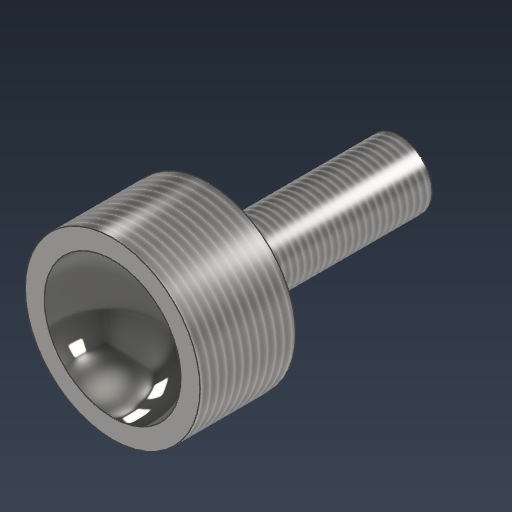
# Autodesk Inventor part: MCEN4000:T1
Saved by Autodesk Inventor 2021 (Build 250183000, 183)
## iProperties
Created: 2020-10-15
Part Number: MCEN4000:T1
Material: STEEL, AISI 1040
Document SubType Name: Modeling
Designer: Eugene Tang
Mass: 109.446 g
Surface Area: 51.7813 cm^2
Volume: 13.9421 cm^3
Density: 7.85 g/cm^3
Appearance: Semi-Polished(1)
Description: TIE ROD INNER CUP
dv: 1.083 mm
dvBigDIA: 0.135 mm
dt: 0.768 mm
dvSmallDIA: 0.128 mm
MinorDIA: 12.000 mm
Pitch: 1.250 mm
a: 0.052 mm
BallJointBall_Dia: 25.000 mm
BallJointBody_THICKNESS: 3.500 mm
BodyDepth: 5.000 mm
q: 40.000 mm
d84: 32.000 mm
Author: Eugene Tang
Autodesk Inventor part; units mm, degrees
ref_plane "YZ Plane" through (0, 0, 0) normal (1, 0, 0) x (0, 1, 0)
ref_plane "XZ Plane" through (0, 0, 0) normal (0, 1, 0) x (-1, 0, 0)
ref_plane "XY Plane" through (0, 0, 0) normal (0, 0, 1) x (1, 0, 0)
sketch "Sketch1" plane through (0, 0, 0) normal (0, 0, 1) x (1, 0, 0)
  circle A0 centre (0, 0) radius 13
  dimension "d0" = 26
  constraints: 1 centre point, 1 coincident
  measures "d0" diameter of A0
sketch "Sketch2" plane through (0, 0, 0) normal (0, 0, 1) x (1, 0, 0)
  circle A0 centre (0, 0) radius 6
  dimension "MinorDIA" = 12
  constraints: 1 centre point, 1 coincident
  measures "MinorDIA" diameter of A0
extrude "Extrusion1" add sketch "Sketch2" against normal blind 40
sketch "Sketch4" plane through (0, 0, 0) normal (1, 0, 0) x (0, 1, 0)
  line L0 (0, 0) -> (0, 25) construction
  circle A0 centre (0, 12.5) radius 12.5 construction
  line L1 (6, 0) -> (-6, 0) projected
  line L2 (6, 0) -> (-6, 0) projected
  line L3 (-16, 12.5) -> (-12.5, 12.5)
  line L4 (-16, 12.5) -> (-16, -5)
  line L5 (-16, -5) -> (0, -5)
  line L6 (0, -5) -> (0, 0)
  line L7 (-12.5, 27.5) -> (-12.5, -3.4028) construction
  arc A1 (-12.5, 12.5) -> (0, 0) centre (0, 12.5) ccw
  dimension "BallJointBall_Dia" = 25
  dimension "BodyDepth" = 5
  dimension "BallJointBody_THICKNESS" = 3.5
  dimension "d52" = 17.5
  constraints: 12 end point, 4 point on circle, 3 tangent, 3 vertical, 2 centre point, 2 perpendicular, 1 horizontal, 1 midpoint, 1 point on line
  measures "BallJointBall_Dia" diameter of A0
  measures "BodyDepth" distance between parallel lines of L5 L1
  measures "BallJointBody_THICKNESS" distance between parallel lines of L4 L7
  measures "d52" distance between parallel lines of L5 L3
revolve "Revolution1" add sketch "Sketch4" angle 360 about axis through (0, 0, 0) along (0, 0, 1)
sketch "Sketch5" plane through (0, 0, 0) normal (1, 0, 0) x (0, 1, 0)
  line L0 (-6, -40) -> (6, -40) construction
  line L1 (6, -40) -> (6, -47.8199) construction
  line L2 (7.0825, -39.5608) -> (7.0825, -47.5953) construction
  line L3 (6.9472, -42.5792) -> (6.9472, -40) construction
  line L4 (6.1797, -43.2466) -> (6.1797, -39.9527) construction
  line L5 (7.0825, -40.625) -> (6, -40.625) construction
  line L6 (6.1279, -41.25) -> (6.1279, -40) construction
  line L7 (6, -40) -> (7.0825, -40) construction
  line L8 (6, -41.25) -> (7.0825, -41.25) construction
  line L9 (7.0825, -40) -> (6, -40.625) construction
  line L10 (6, -40.625) -> (7.0825, -41.25) construction
  arc A0 (6.1797, -40.5213) -> (6.1797, -40.7287) centre (6.2578, -40.625) ccw
  line L11 (6.9472, -40) -> (6.9472, -40.0781)
  line L12 (6.9472, -40.0781) -> (6.1797, -40.5213)
  line L13 (6.9472, -41.1719) -> (6.9472, -41.25)
  line L14 (6.9472, -41.1719) -> (6.1797, -40.7287)
  line L15 (6.9472, -40.0781) -> (6.9472, -41.1719)
  point P0 (0, 0)
  dimension "dv" = 1.0825
  dimension "dvBigDIA" = 0.1353
  dimension "dt" = 0.7675
  dimension "d12" = 1.25
  dimension "d13" = 0.625
  dimension "dvSmallDIA" = 0.1279
  dimension "d16" = 0.9472
  dimension "d19" = 59.999
  dimension "d22" = 0.5469
  dimension "a" = 0.0518
  constraints: 30 end point, 18 point on line, 3 perpendicular, 3 vertical, 2 collinear, 2 parallel, 2 point on circle, 1 centre point, 1 tangent
  measures "dv" distance between parallel lines of L1 L2
  measures "dvBigDIA" distance between parallel lines of L2 L3
  measures "dt" distance between parallel lines of L3 L4
  measures "d12" distance of L0.end L8.start
  measures "d13" distance from line of L8.start L5
  measures "dvSmallDIA" distance between parallel lines of L6 L1
  measures "d16" distance between parallel lines of L3 L1
  measures "d19" angle of L1 L9
  measures "d22" distance from line of L11.end L5
  measures "a" distance between parallel lines of L6 L4
thread "Thread5" size "M12x1.25" class "6g" standard "ISO Metric profile" full length
thread "Thread6" size "M32x1.5" class "6g" standard "ISO Metric profile" full length
sketch "Sketch13" plane through (0, 0, 12.5) normal (0, 0, 1) x (1, 0, 0)
  circle A0 centre (0, 0) radius 16 projected
  dimension "d84" = 32
  measures "d84" diameter of A0
equation "\"d0\" = SteeringColumn_DIA"
equation "\"dv\" = 0.866 * Pitch"
equation "\"dvBigDIA\" = 0.125 * dv"
equation "\"dt\" = 0.614 * Pitch"
equation "\"d12\" = Pitch"
equation "\"d13\" = 0.5 * d12"
equation "\"dvSmallDIA\" = 0.166667 * dt"
equation "\"TD\" = 0.3"
equation "\"Ball_DIA\" = 6"
equation "\"Screw_L\" = 292"
equation "\"Screw_DIA\" = 36"
equation "\"Nut_OD\" = 66"
equation "\"BPath_REVQ\" = 5.75"
equation "\"Tread_OFFSET\" = 8.075"
equation "\"SteeringColumn_DIA\" = 26"
equation "\"SteeringColumnChamfer_DEG\" = 20deg"
equation "\"Rack_L\" = 307.252"
equation "\"Pitch\" = 1.25"
equation "\"NutCapTread_L\" = 25"
equation "\"NutCapTread_THICKNESS\" = 5.365"
equation "\"NutCap_THICKNESS\" = 5.38"
equation "\"GearToHub_Ratio\" = 0.6"
equation "\"SupportFlange_THICKNESS\" = 5"
equation "\"GearKey_L\" = 32"
body "Solid1"
